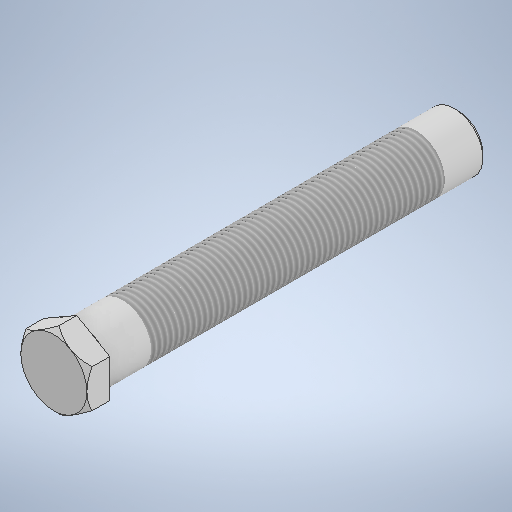
# Autodesk Inventor part: Main Bolt
Saved by Autodesk Inventor 2025.2 (Build 292293000, 293)
## iProperties
Created: 2025-02-09
Part Number: Main Bolt
Material: Generic
Document SubType Name: Modeling
Designer: mpava
Density: 1 g/cm^3
Appearance: Default
Author: mpava
Autodesk Inventor part; units mm, degrees
ref_plane "YZ Plane" through (0, 0, 0) normal (1, 0, 0) x (0, 1, 0)
ref_plane "XZ Plane" through (0, 0, 0) normal (0, 1, 0) x (-1, 0, 0)
ref_plane "XY Plane" through (0, 0, 0) normal (0, 0, 1) x (1, 0, 0)
sketch "Sketch1" plane through (0, 0, 0) normal (0, 0, 1) x (1, 0, 0)
  line L0 (8.6603, -5) -> (0, -10)
  line L1 (0, -10) -> (-8.6603, -5)
  line L2 (-8.6603, -5) -> (-8.6603, 5)
  line L3 (-8.6603, 5) -> (0, 10)
  line L4 (0, 10) -> (8.6603, 5)
  line L5 (8.6603, 5) -> (8.6603, -5)
  point P0 (0, 0)
  point P1 (0, 0)
  dimension "d0" = 10
  constraints: 12 end point, 1 coincident, 1 vertical, 13 other
  measures "d0" distance of L1.end L2.end
extrude "Extrusion1" add sketch "Sketch1" along normal blind 6
sketch "Sketch2" plane through (0, 0, 6) normal (0, 0, 1) x (1, 0, 0)
  circle A0 centre (0, 0) radius 8.6603
  line L0 (0, -10) -> (8.6603, -5) projected
  constraints: 1 centre point, 1 coincident, 1 tangent
extrude "Extrusion2" cut sketch "Sketch2" against normal blind 6 draft 45 keep common part
sketch "Sketch3" plane through (0, 0, 0) normal (0, 0, -1) x (-1, 0, 0)
  circle A0 centre (0, 0) radius 7.5
  dimension "d5" = 15
  constraints: 1 centre point, 1 coincident
  measures "d5" diameter of A0
extrude "Extrusion3" add sketch "Sketch3" along normal blind 100
fillet "Fillet1" radius 1 1 edges at (7.5, 0, 0)
chamfer "Chamfer1" distance 1 angle 45 1 edges at (7.5, 0, -100)
sketch "Sketch4" plane through (0, 0, 0) normal (0, 1, 0) x (-1, 0, 0)
  point P0 (0, 0)
sketch "Sketch5" plane through (0, 0, 0) normal (0, 1, 0) x (-1, 0, 0)
  point P0 (0, 0)
thread "Thread1" size "M15x1.5" class "6g" standard "ANSI Metric M Profile" length 77 offset 11
body "Solid1"
